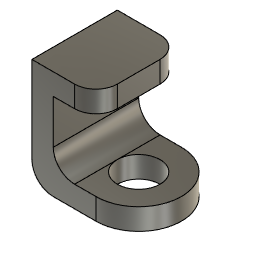
Exercise_03 (Autodesk Fusion 360 design; units mm, degrees)
Autodesk Fusion 360 part; units mm, degrees
sketch "Sketch1" plane through (0, 0, 0) normal (0, 1, 0) x (1, 0, 0)
  line L0 (29.7004, -65.6) -> (29.7004, -55.6)
  line L1 (29.7004, -55.6) -> (9.7004, -55.6)
  line L2 (9.7004, -55.6) -> (9.7004, -25)
  line L3 (9.7004, -25) -> (29.7004, -25)
  line L4 (29.7004, -25) -> (29.7004, -15)
  line L5 (29.7004, -15) -> (-0.2996, -15)
  line L6 (-0.2996, -15) -> (-0.2996, -65.6)
  line L7 (-0.2996, -65.6) -> (29.7004, -65.6)
  dimension "d1" = 10
  dimension "d2" = 10
  dimension "d5" = 10
  dimension "d6" = 30
  dimension "d7" = 50.6
  dimension "d8" = 30
  constraint vertical L0
  constraint perpendicular L0 L1
  constraint perpendicular L1 L2
  constraint perpendicular L0 L3
  constraint perpendicular L1 L4
  constraint perpendicular L0 L5
  constraint perpendicular L1 L6
  constraint perpendicular L0 L7
  measures "d1" distance of L0.start L0.end
  measures "d2" distance of L3.end L4.end
  measures "d5" distance of L2 L6
  measures "d6" distance of L0.start L6.end
  measures "d7" distance of L5.end L6.end
  measures "d8" distance of L4.end L5.end
extrude "Extrude1" add sketch "Sketch1" along normal blind 40
sketch "Sketch2" plane through (0, 0, 15) normal (0, 0, -1) x (1, 0, 0)
  line L0 (29.7004, 0) -> (-0.2996, 0)
  line L1 (-0.2996, 0) -> (-0.2996, -40)
  line L2 (-0.2996, -40) -> (29.7004, -40)
  line L3 (29.7004, -40) -> (29.7004, 0)
  circle A0 centre (29.7004, -20) radius 20
  circle A1 centre (29.7004, -20) radius 10
  dimension "d11" = 20
  constraint midpoint L3 A0.centre
  constraint coincident L0.start A0
  constraint concentric A0 A1
  measures "d11" diameter of A1
extrude "Extrude2" add sketch "Sketch2" against normal blind 10 contours L3 A0 A1 picked at (46.2992, -20.9488)
extrude "Extrude3" cut sketch "Sketch2" against normal blind 10 contours L3 A1 picked at (26.4507, -19.2583)
fillet "Fillet1" radius 10 1 edges at (-0.2996, 20, 15)
fillet "Fillet2" radius 10 1 edges at (9.7004, 20, 25)
fillet "Fillet3" radius 10 2 edges at (29.7004, 0, 60.6) (29.7004, 40, 60.6)
